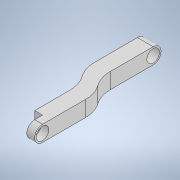
# Autodesk Inventor part: Рулевая тяга
Saved by Autodesk Inventor 2020 (Build 240168000, 168)
## iProperties
Created: 2021-07-18
Part Number: Рулевая тяга
Material: Типовые
Document SubType Name: Modeling
Designer: Антон
Density: 1 g/cm^3
Appearance: По умолчанию
Author: Антон
Autodesk Inventor part; units mm, degrees
ref_plane "YZ Plane" through (0, 0, 0) normal (1, 0, 0) x (0, 1, 0)
ref_plane "XZ Plane" through (0, 0, 0) normal (0, 1, 0) x (-1, 0, 0)
ref_plane "XY Plane" through (0, 0, 0) normal (0, 0, 1) x (1, 0, 0)
sketch "Эскиз1" plane through (0, 0, 0) normal (0, 1, 0) x (-1, 0, 0)
  line L0 (0, 0) -> (4, 0)
  line L1 (4, 0) -> (4, -19.536)
  line L2 (4, -19.536) -> (0, -19.536)
  line L3 (0, -19.536) -> (0, 0)
  line L4 (0, -19.536) -> (7, -19.536)
  line L5 (7, -19.536) -> (7, -15.536)
  line L6 (7, -15.536) -> (0, -15.536)
  line L7 (0, -15.536) -> (0, -19.536)
  line L8 (7, -15.536) -> (3, -15.536)
  line L9 (3, -15.536) -> (3, -35.072)
  line L10 (3, -35.072) -> (7, -35.072)
  line L11 (7, -35.072) -> (7, -15.536)
  line L12 (2, 0) -> (2, -2) construction
  line L13 (5, -35.072) -> (5, -33.072) construction
  line L14 (7, -19.536) -> (4, -15.536)
  line L15 (0, -15.536) -> (3, -19.536)
  point P0 (4, -15.536)
  point P1 (7, -19.536)
  dimension "d10" = 4
  dimension "d11" = 7
  dimension "d15" = 2
  dimension "d17" = 31.072
  constraints: 32 end point, 6 parallel, 4 equal length, 4 point on line, 3 horizontal, 3 perpendicular, 2 midpoint, 2 vertical
  measures "d10" distance of L0.start L0.end
  measures "d11" distance between parallel lines of L3 L11
  measures "d15" distance of L12.start L12.end
  measures "d17" vertical distance of L12.end L13.end
extrude "Выдавливание1" add sketch "Эскиз1" along normal blind 4 contours L0 L1 L6 L3 | L6 L9 L15 | L14 L4 L1 | L1 L2 L9 L6 | L2 L4 L11 L10 L9
fillet "Сопряжение2" radius 8 4 edges at (-7, 2, -19.536) (-4, 2, -15.536) (0, 2, -15.536) (-3, 2, -19.536)
sketch "Эскиз3" plane through (-7, 0, 1.2) normal (-1, 0, 0) x (0, 0, 1)
  line L0 (-1.2, 0) -> (-1.2, 4) projected
  line L1 (-1.2, 2) -> (-3.2, 2)
  line L2 (-36.272, 0) -> (-36.272, 4) projected
  line L3 (-36.272, 2) -> (-34.272, 2)
  dimension "d18" = 2
  constraints: 4 end point, 2 horizontal, 2 midpoint, 1 collinear
  measures "d18" distance of L1.start L1.end
hole "Отверстие1" at (-7, 2, -2) at (-7, 2, -33.072) direction (1, 0, 0) diameter 3.2 end through all
fillet "Сопряжение3" radius 2 4 edges at (-2, 4, 0) (-2, 0, 0) (-5, 4, -35.072) (-5, 0, -35.072)
sketch "Эскиз5" plane through (-4, 0, -12.8753) normal (-1, 0, 0) x (0, 0, 1)
  circle A0 centre (10.8753, 2) radius 1.6 projected
  circle A1 centre (10.8753, 2) radius 2
  arc A2 (10.8753, 0) -> (10.8753, 4) centre (10.8753, 2) ccw projected
  line L0 (10.8753, 4) -> (0, 4) projected
  line L1 (12.8753, 0) -> (8.8753, 0)
  line L2 (8.8753, 0) -> (8.8753, 4)
  line L3 (8.8753, 4) -> (12.8753, 4)
  line L4 (12.8753, 4) -> (12.8753, 0)
  line L5 (12.8753, 0) -> (8.8753, 4) construction
  line L6 (8.8753, 0) -> (12.8753, 4) construction
  point P0 (12.8753, 0)
  point P1 (8.8753, 2)
  point P2 (10.8753, 0)
  point P3 (10.8753, 4)
  constraints: 12 end point, 2 midpoint, 2 parallel, 2 perpendicular, 1 centre point, 1 coincident, 1 concentric, 1 horizontal, 1 point on line
extrude "Выдавливание3" cut sketch "Эскиз5" against normal blind 2 contours A0 | A1 | A1 L2 L0 | L1 L2 A1
